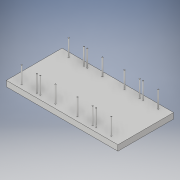
# Autodesk Inventor part: Part4
Saved by Autodesk Inventor 2018 (Build 220112000, 112)
## iProperties
Created: 2017-12-28
Part Number: Part4
Material: Generic
Document SubType Name: Modeling
Designer: BB-8
Density: 1 g/cm^3
Appearance: Default
Author: BB-8
Autodesk Inventor part; units mm, degrees
ref_plane "YZ Plane" through (0, 0, 0) normal (1, 0, 0) x (0, 1, 0)
ref_plane "XZ Plane" through (0, 0, 0) normal (0, 1, 0) x (-1, 0, 0)
ref_plane "XY Plane" through (0, 0, 0) normal (0, 0, 1) x (1, 0, 0)
sketch "Sketch1" plane through (0, 0, 0) normal (0, 1, 0) x (-1, 0, 0)
  line L0 (0, 0) -> (200, 0)
  line L1 (200, 0) -> (200, -100)
  line L2 (200, -100) -> (0, -100)
  line L3 (0, -100) -> (0, 0)
  circle A0 centre (19.68, -7.9) radius 1
  circle A1 centre (46.98, -7.9) radius 1
  circle A2 centre (80.31, -7.9) radius 1
  circle A3 centre (53.01, -7.9) radius 1
  circle A4 centre (19.68, -92.1) radius 1
  circle A5 centre (46.98, -92.1) radius 1
  circle A6 centre (80.31, -92.1) radius 1
  circle A7 centre (53.01, -92.1) radius 1
  circle A8 centre (180.32, -7.9) radius 1
  circle A9 centre (153.02, -7.9) radius 1
  circle A10 centre (119.69, -7.9) radius 1
  circle A11 centre (146.99, -7.9) radius 1
  circle A12 centre (119.69, -92.1) radius 1
  circle A13 centre (146.99, -92.1) radius 1
  circle A14 centre (153.02, -92.1) radius 1
  circle A15 centre (180.32, -92.1) radius 1
  point P0 (33.33, 0)
  point P1 (33.33, -7.9)
  dimension "d0" = 200
  dimension "d1" = 100
  dimension "d5" = 2
  dimension "d6" = 2
  dimension "d9" = 2
  dimension "d10" = 2
  constraints: 16 centre point, 8 end point, 2 parallel, 1 horizontal, 1 perpendicular, 1 point on line
  measures "d0" distance of L1.end L2.end
  measures "d1" distance of L0.end L1.end
  measures "d5" diameter of A0
  measures "d6" diameter of A1
  measures "d9" diameter of A2
  measures "d10" diameter of A3
extrude "Extrusion1" add sketch "Sketch1" along normal blind 30 contours A0 | A1 | A2 | A3
extrude "Extrusion2" add sketch "Sketch1" along normal blind 30 contours A4 | A5 | A6 | A7 | A8 | A9 | A10 | A11 | A12 | A13 | A14 | A15
extrude "Extrusion3" add sketch "Sketch1" against normal blind 10
body "Solid1"
